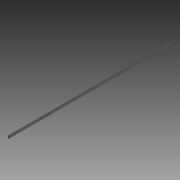
# Autodesk Inventor part: X_Rai-SquareBar-Rev3
Saved by Autodesk Inventor 2015 (Build 190159000, 159)
## iProperties
Created: 2017-01-08
Part Number: X_Rai-SquareBar-Rev3
Material: Iron, Ductile
Document SubType Name: Modeling
Designer: Guy
Density: 7.15 g/cm^3
Appearance: Iron Gray
Author: Guy
Autodesk Inventor part; units mm, degrees
ref_plane "YZ Plane" through (0, 0, 0) normal (1, 0, 0) x (0, 1, 0)
ref_plane "XZ Plane" through (0, 0, 0) normal (0, 1, 0) x (-1, 0, 0)
ref_plane "XY Plane" through (0, 0, 0) normal (0, 0, 1) x (1, 0, 0)
sketch "Sketch1" plane through (0, 0, 0) normal (0, 0, 1) x (1, 0, 0)
  line L0 (0, 0) -> (6.35, 0)
  line L1 (6.35, 0) -> (6.35, 38.1)
  line L2 (6.35, 38.1) -> (0, 38.1)
  line L3 (0, 38.1) -> (0, 0)
  dimension "d0" = 6.35
  dimension "d1" = 38.1
  constraints: 8 end point, 2 parallel, 1 horizontal, 1 perpendicular
  measures "d0" distance between parallel lines of L3 L1
  measures "d1" distance between parallel lines of L0 L2
extrude "Extrusion1" add sketch "Sketch1" along normal blind 2700
sketch "Sketch2" plane through (6.35, 38.1, 2700) normal (1, 0, 0) x (0, 0, -1)
  line L0 (2700, -38.1) -> (2700, 0) projected
  line L1 (2700, 0) -> (0, 0) projected
  line L2 (0, -38.1) -> (0, 0) projected
  line L3 (2700, -38.1) -> (0, -38.1) projected
  circle A0 centre (550, -19.05) radius 6.35
  circle A1 centre (750, -19.05) radius 6.35
  circle A2 centre (950, -19.05) radius 6.35
  circle A3 centre (1750, -19.05) radius 6.35
  circle A4 centre (1950, -19.05) radius 6.35
  circle A5 centre (2150, -19.05) radius 6.35
  dimension "d4" = 12.7
  dimension "d5" = 19.05
  dimension "d6" = 12.7
  dimension "d7" = 12.7
  dimension "d8" = 12.7
  dimension "d9" = 12.7
  dimension "d10" = 12.7
  dimension "d11" = 550
  dimension "d12" = 200
  dimension "d13" = 200
  dimension "d14" = 550
  dimension "d15" = 200
  dimension "d16" = 200
  dimension "d17" = 19.05
  dimension "d18" = 19.05
  dimension "d19" = 19.05
  dimension "d20" = 19.05
  dimension "d21" = 19.05
  constraints: 6 centre point
  measures "d4" diameter of A0
  measures "d5" distance from line of L3 A0.centre
  measures "d6" diameter of A1
  measures "d7" diameter of A2
  measures "d8" diameter of A3
  measures "d9" diameter of A4
  measures "d10" diameter of A5
  measures "d11" distance from line of A0.centre L2
  measures "d12" distance of A0.centre A1.centre
  measures "d13" distance of A1.centre A2.centre
  measures "d14" distance from line of L0 A5.centre
  measures "d15" distance of A4.centre A5.centre
  measures "d16" distance of A3.centre A4.centre
  measures "d17" distance from line of L3 A1.centre
  measures "d18" distance from line of L3 A2.centre
  measures "d19" distance from line of A3.centre L3
  measures "d20" distance from line of L3 A4.centre
  measures "d21" distance from line of L3 A5.centre
extrude "Extrusion3" cut sketch "Sketch2" against normal blind 10 contours A0 | A1 | A2 | A3 | A4 | A5
sketch "Sketch3" plane through (0, 0, 0) normal (-1, 0, 0) x (0, 0, 1)
  circle A0 centre (750, 19.05) radius 6.35 projected
  circle A1 centre (1750, 19.05) radius 6.35 projected
  circle A2 centre (2150, 19.05) radius 6.35 projected
  circle A3 centre (1950, 19.05) radius 6.35 projected
  circle A4 centre (950, 19.05) radius 6.35 projected
  circle A5 centre (550, 19.05) radius 6.35 projected
  line L0 (0, 38.1) -> (0, 0) projected
  line L1 (0, 0) -> (2700, 0) projected
  line L2 (2700, 38.1) -> (2700, 0) projected
  line L3 (0, 38.1) -> (2700, 38.1) projected
  circle A6 centre (2658.6, 12.5) radius 4
  circle A7 centre (2685, 12.5) radius 4
  dimension "d26" = 8
  dimension "d27" = 8
  dimension "d28" = 12.5
  dimension "d29" = 12.5
  dimension "d30" = 15
  dimension "d31" = 26.4
  constraints: 2 centre point
  measures "d26" diameter of A7
  measures "d27" diameter of A6
  measures "d28" distance from line of L1 A6.centre
  measures "d29" distance from line of L1 A7.centre
  measures "d30" distance from line of A7.centre L2
  measures "d31" distance of A7.centre A6.centre
extrude "Extrusion4" cut sketch "Sketch3" against normal blind 10 contours A6 | A7
sketch "Sketch5" plane through (6.35, 38.1, 2700) normal (1, 0, 0) x (0, 0, -1)
  circle A0 centre (2680, -12.5) radius 4
  circle A1 centre (2680, -27.5) radius 4
  circle A2 centre (41.4, -25.6) radius 4 projected
  circle A3 centre (15, -25.6) radius 4 projected
  circle A4 centre (1950, -19.05) radius 6.35 projected
  circle A5 centre (950, -19.05) radius 6.35 projected
  circle A6 centre (550, -19.05) radius 6.35 projected
  circle A7 centre (750, -19.05) radius 6.35 projected
  circle A8 centre (1750, -19.05) radius 6.35 projected
  circle A9 centre (2150, -19.05) radius 6.35 projected
  line L0 (2700, -38.1) -> (2700, 0) projected
  line L1 (2700, 0) -> (0, 0) projected
  line L2 (0, -38.1) -> (0, 0) projected
  line L3 (2700, -38.1) -> (0, -38.1) projected
  dimension "d49" = 8
  dimension "d50" = 8
  dimension "d51" = 20
  dimension "d52" = 20
  dimension "d53" = 12.5
  dimension "d54" = 15
  constraints: 2 centre point
  measures "d49" diameter of A0
  measures "d50" diameter of A1
  measures "d51" distance from line of A0.centre L0
  measures "d52" distance from line of L0 A1.centre
  measures "d53" distance from line of L1 A0.centre
  measures "d54" distance of A1.centre A0.centre
extrude "Extrusion6" cut sketch "Sketch5" against normal up to next contours A0 | A1
body "Solid1"
